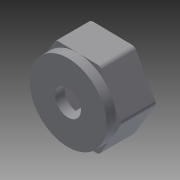
# Autodesk Inventor part: MagnetHolder 6mm
Saved by Autodesk Inventor 2014 (Build 180170000, 170)
## iProperties
Created: 2014-01-11
Part Number: MagnetHolder 6mm
Material: Generic
Document SubType Name: Modeling
Designer: intern
Density: 1 g/cm^3
Appearance: Default
Author: intern
Autodesk Inventor part; units mm, degrees
ref_plane "YZ Plane" through (0, 0, 0) normal (1, 0, 0) x (0, 1, 0)
ref_plane "XZ Plane" through (0, 0, 0) normal (0, 1, 0) x (-1, 0, 0)
ref_plane "XY Plane" through (0, 0, 0) normal (0, 0, 1) x (1, 0, 0)
sketch "Sketch2" plane through (0, 0, 0) normal (0, 0, 1) x (1, 0, 0)
  line L0 (3.7629, 6.2932) -> (-3.5686, 6.4054) projected
  line L1 (-3.5686, 6.4054) -> (-7.3315, 0.1122) projected
  line L2 (-7.3315, 0.1122) -> (-3.7629, -6.2932) projected
  line L3 (-3.7629, -6.2932) -> (3.5686, -6.4054) projected
  line L4 (3.5686, -6.4054) -> (7.3315, -0.1122) projected
  line L5 (7.3315, -0.1122) -> (3.7629, 6.2932) projected
  line L6 (3.5686, -6.4054) -> (-3.5686, 6.4054)
  line L7 (-3.5686, 6.4054) -> (-5.0286, 9.0261)
  line L8 (7.3315, -0.1122) -> (-7.3315, 0.1122)
  line L9 (-5.0286, 9.0261) -> (5.3025, 8.868)
  line L10 (5.3025, 8.868) -> (10.3311, -0.1581)
  line L11 (10.3311, -0.1581) -> (5.0286, -9.0261)
  line L12 (5.0286, -9.0261) -> (-5.3025, -8.868)
  line L13 (-5.3025, -8.868) -> (-10.3311, 0.1581)
  line L14 (-10.3311, 0.1581) -> (-5.0286, 9.0261)
  line L15 (-3.5686, 6.4054) -> (3.7629, 6.2932)
  line L16 (3.7629, 6.2932) -> (7.3315, -0.1122)
  line L17 (7.3315, -0.1122) -> (3.5686, -6.4054)
  line L18 (3.5686, -6.4054) -> (-3.7629, -6.2932)
  line L19 (-3.7629, -6.2932) -> (-7.3315, 0.1122)
  line L20 (-7.3315, 0.1122) -> (-3.5686, 6.4054)
  point P0 (0, 0)
  point P1 (0, 0)
  point P2 (0, 0)
  dimension "d0" = 3
  constraints: 30 end point, 2 coincident, 2 parallel, 1 collinear, 26 other
  measures "d0" distance of L0.end L7.end
extrude "Extrusion1" add sketch "Sketch2" against normal blind 8
sketch "Sketch3" plane through (0, 0, 0) normal (0, 0, 1) x (1, 0, 0)
  line L0 (-5.0286, 9.0261) -> (-10.3311, 0.1581) projected
  line L1 (-5.3025, -8.868) -> (5.0286, -9.0261) projected
  line L2 (10.3311, -0.1581) -> (5.3025, 8.868) projected
  circle A0 centre (0, 0) radius 8.9481
  circle A1 centre (0, 0) radius 3
  point P0 (0, 0)
  dimension "d3" = 6
  constraints: 3 tangent, 2 centre point, 1 coincident
  measures "d3" diameter of A1
extrude "Extrusion2" add sketch "Sketch3" along normal blind 2.2
fillet "Fillet1" radius 1 6 edges at (-5.3025, -8.868, -4) (-10.3311, 0.1581, -4) (-5.0286, 9.0261, -4) (5.3025, 8.868, -4) (10.3311, -0.1581, -4) (5.0286, -9.0261, -4)
body "Solid1"
